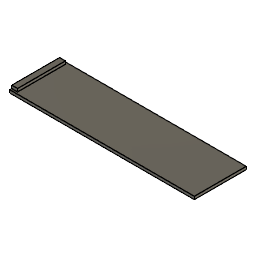
Canal - top plate v3 (Autodesk Fusion 360 design; units mm, degrees)
Autodesk Fusion 360 part; units mm, degrees
sketch "Esquisse1" plane through (0, 0, 0) normal (0, 0, 1) x (1, 0, 0)
  line L0 (4.3054, 30) -> (67.3054, 30)
  line L1 (67.3054, 30) -> (67.3054, 12.25)
  line L2 (67.3054, 12.25) -> (4.3054, 12.25)
  line L3 (4.3054, 12.25) -> (4.3054, 30)
  dimension "d1" = 63
  dimension "d2" = 17.75
  constraint horizontal L0
  constraint vertical L1
  constraint horizontal L2
  constraint vertical L3
  measures "d1" distance of L1 L3
  measures "d2" distance of L0 L2
extrude "Extrusion1" add sketch "Esquisse1" along normal blind 1
sketch "Esquisse2" plane through (0, 0, 1) normal (0, 0, 1) x (-1, 0, 0)
  line L0 (-4.3054, -12.25) -> (-67.3054, -12.25)
  line L1 (-67.3054, -12.25) -> (-67.3054, -30)
  line L2 (-67.3054, -30) -> (-4.3054, -30)
  line L3 (-4.3054, -30) -> (-4.3054, -12.25)
  line L4 (-4.3054, -12.95) -> (-6.3054, -12.95)
  line L5 (-6.3054, -12.95) -> (-6.3054, -29.3)
  line L6 (-6.3054, -29.3) -> (-4.3054, -29.3)
  line L7 (-4.3054, -29.3) -> (-4.3054, -12.95)
  line L8 (-67.3054, -21.125) -> (-4.3054, -21.125) construction
  dimension "d5" = 16.35
  dimension "d8" = 2
  constraint horizontal L4
  constraint vertical L5
  constraint horizontal L6
  constraint vertical L7
  constraint coincident L3 L4.start
  constraint midpoint L1 L8.start
  constraint midpoint L3 L8.end
  constraint symmetric L4 L6 L8
  measures "d5" distance of L4.end L5.end
  measures "d8" distance of L5.end L6.end
extrude "Extrusion2" add sketch "Esquisse2" along normal blind 1 contours L3 L4 L5 L6 L7
